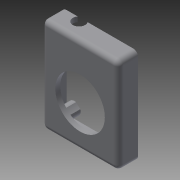
# Autodesk Inventor part: rounded_top
Saved by Autodesk Inventor 2014 SP1 (Build 180222100, 222)
## iProperties
Created: 2016-10-19
Part Number: rounded_top
Material: Generic
Document SubType Name: Modeling
Designer: danielsikar
Density: 1 g/cm^3
Appearance: Default
Author: danielsikar
Autodesk Inventor part; units mm, degrees
ref_plane "YZ Plane" through (0, 0, 0) normal (1, 0, 0) x (0, 1, 0)
ref_plane "XZ Plane" through (0, 0, 0) normal (0, 1, 0) x (-1, 0, 0)
ref_plane "XY Plane" through (0, 0, 0) normal (0, 0, 1) x (1, 0, 0)
sketch "Sketch1" plane through (0, 0, 0) normal (0, 1, 0) x (-1, 0, 0)
  line L0 (0, 0) -> (30.9, 0)
  line L1 (30.9, 0) -> (30.9, 38.5)
  line L2 (30.9, 38.5) -> (0, 38.5)
  line L3 (0, 38.5) -> (0, 0)
  dimension "d0" = 30.9
  dimension "d1" = 38.5
  constraints: 8 end point, 2 parallel, 1 horizontal, 1 perpendicular
  measures "d0" distance of L2.end L1.end
  measures "d1" distance between parallel lines of L0 L2
extrude "Extrusion1" add sketch "Sketch1" along normal blind 2
sketch "Sketch2" plane through (0, 2, 0) normal (0, 1, 0) x (1, 0, 0)
  line L0 (-30.9, 0) -> (-30.9, -38.5) projected
  line L1 (-30.9, -38.5) -> (0, -38.5) projected
  circle A0 centre (-23.7, -7.8) radius 1.5
  circle A1 centre (-7.2, -7.8) radius 1.5
  circle A2 centre (-15.45, -16.7) radius 10
  dimension "d4" = 3
  dimension "d5" = 3
  dimension "d6" = 30.7
  dimension "d7" = 30.7
  dimension "d8" = 7.2
  dimension "d9" = 16.5
  dimension "d30" = 20
  dimension "d31" = 15.45
  dimension "d32" = 21.8
  constraints: 3 centre point
  measures "d4" diameter of A0
  measures "d5" diameter of A1
  measures "d6" distance from line of L1 A0.centre
  measures "d7" distance from line of L1 A1.centre
  measures "d8" distance from line of A0.centre L0
  measures "d9" distance of A1.centre A0.centre
  measures "d30" diameter of A2
  measures "d31" distance from line of A2.centre L0
  measures "d32" distance from line of A2.centre L1
sketch "Sketch5" plane through (0, 2, 0) normal (0, 1, 0) x (1, 0, 0)
  line L0 (-30.9, 0) -> (-30.9, -38.5) projected
  line L1 (-30.9, -38.5) -> (0, -38.5) projected
  line L2 (-30.9, 0) -> (0, 0)
  line L3 (0, 0) -> (0, -38.5)
  line L4 (0, -38.5) -> (-30.9, -38.5)
  line L5 (-30.9, -38.5) -> (-30.9, 0)
  line L6 (-28.9, -2) -> (-2, -2)
  line L7 (-2, -2) -> (-2, -36.5)
  line L8 (-2, -36.5) -> (-28.9, -36.5)
  line L9 (-28.9, -36.5) -> (-28.9, -2)
  dimension "d18" = 26.9
  dimension "d19" = 34.5
  dimension "d20" = 2
  dimension "d21" = 2
  constraints: 16 end point, 4 parallel, 2 horizontal, 2 perpendicular
  measures "d18" distance of L7.end L8.end
  measures "d19" distance of L6.end L7.end
  measures "d20" distance between parallel lines of L1 L8
  measures "d21" distance between parallel lines of L9 L0
extrude "Extrusion5" add sketch "Sketch5" along normal blind 6
fillet "Fillet1" radius 2 8 edges at (0, 4, 38.5) (-30.9, 4, 38.5) (0, 4, 0) (-30.9, 4, 0) (-15.45, 0, 38.5) (-30.9, 0, 19.25) (0, 0, 19.25) (-15.45, 0, 0)
extrude "Extrusion7" cut sketch "Sketch2" against normal blind 2
sketch "Sketch7" plane through (0, 2, 0) normal (0, 1, 0) x (1, 0, 0)
  circle A0 centre (-7.2, -7.8) radius 1.5 projected
  circle A1 centre (-23.7, -7.8) radius 1.5 projected
  circle A2 centre (-15.45, -16.7) radius 10 projected
  circle A3 centre (-23.7, -7.8) radius 1.5
  circle A4 centre (-7.2, -7.8) radius 1.5
  arc A5 (-21.3371, -8.6166) -> (-23.0646, -10.2179) centre (-23.7, -7.8) ccw
  arc A6 (-7.8354, -10.2179) -> (-9.5629, -8.6166) centre (-7.2, -7.8) ccw
  arc A7 (-21.3371, -8.6166) -> (-23.0646, -10.2179) centre (-15.45, -16.7) ccw
  arc A8 (-7.8354, -10.2179) -> (-9.5629, -8.6166) centre (-15.45, -16.7) ccw
  point P0 (0, 0)
  dimension "d35" = 5
  dimension "d36" = 5
  constraints: 8 point on circle, 6 centre point, 5 coincident, 2 concentric
  measures "d35" diameter of A5
  measures "d36" diameter of A6
extrude "Extrusion8" add sketch "Sketch7" along normal blind 4 contours A2 A6 | A5 A2
sketch "Sketch8" plane through (0, 0, 0) normal (0, -1, 0) x (1, 0, 0)
  circle A0 centre (-7.2, 7.8) radius 1.5 projected
  circle A1 centre (-23.7, 7.8) radius 1.5 projected
  circle A2 centre (-23.7, 7.8) radius 1.5
  circle A3 centre (-7.2, 7.8) radius 1.5
  point P0 (0, 0)
  constraints: 2 centre point, 2 coincident, 2 concentric
extrude "Extrusion9" add sketch "Sketch8" against normal blind 2
sketch "Sketch10" plane through (-28.9, 8, 38.5) normal (0, 0, 1) x (1, 0, 0)
  line L0 (0, 0) -> (26.9, 0) projected
  line L1 (0, -6) -> (0, 0) projected
  circle A0 centre (6.5, -1.5) radius 2.5
  point P0 (28.9, -8)
  dimension "d45" = 5
  dimension "d46" = 6.5
  dimension "d47" = 1.5
  constraints: 1 centre point
  measures "d45" diameter of A0
  measures "d46" distance from line of A0.centre L1
  measures "d47" distance from line of A0.centre L0
extrude "Extrusion11" cut sketch "Sketch10" against normal blind 2
body "Solid1"
